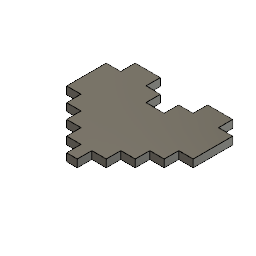
heart (Autodesk Fusion 360 design; units mm, degrees)
Autodesk Fusion 360 part; units mm, degrees
sketch "Sketch1" plane through (0, 0, 0) normal (0, 1, 0) x (1, 0, 0)
  line L0 (-2.775, 16.15) -> (-8.325, 16.15)
  line L1 (2.775, -22.7) -> (2.775, -17.15)
  line L2 (13.875, -11.6) -> (8.325, -11.6)
  line L3 (28.5, -28) -> (28.5, 27)
  line L4 (-2.775, -17.15) -> (-2.775, -22.7)
  line L5 (-2.775, -22.7) -> (2.775, -22.7)
  line L6 (8.325, -17.15) -> (2.775, -17.15)
  line L7 (-28.5, 27) -> (-28.5, -28)
  line L8 (28.5, 27) -> (-28.5, 27)
  line L9 (19.425, -6.05) -> (13.875, -6.05)
  line L10 (-8.325, -17.15) -> (-2.775, -17.15)
  line L11 (28.5, -0.5) -> (-28.5, -0.5)
  line L12 (24.975, -0.5) -> (19.425, -0.5)
  line L13 (19.425, -0.5) -> (19.425, -6.05)
  line L14 (-24.975, 16.15) -> (-24.975, -0.5)
  line L15 (0, 5.05) -> (0, -0.5)
  line L16 (-24.975, -0.5) -> (-19.425, -0.5)
  line L17 (0, 10.6) -> (-2.775, 10.6)
  line L18 (0, 27) -> (0, -28)
  line L19 (24.975, 16.15) -> (24.975, -0.5)
  line L20 (0, -0.5) -> (0, -22.7)
  line L21 (0, -0.5) -> (0, 21.7)
  line L22 (-13.875, -6.05) -> (-13.875, -11.6)
  line L23 (-19.425, -6.05) -> (-13.875, -6.05)
  line L24 (0, 10.6) -> (0, 5.05)
  line L25 (-19.425, -0.5) -> (-19.425, -6.05)
  line L26 (-8.325, -11.6) -> (-8.325, -17.15)
  line L27 (19.425, 21.7) -> (19.425, 16.15)
  line L28 (-19.425, 21.7) -> (-19.425, 16.15)
  line L29 (-13.875, -11.6) -> (-8.325, -11.6)
  line L30 (-8.325, 16.15) -> (-8.325, 21.7)
  line L31 (-2.775, 10.6) -> (-2.775, 16.15)
  line L32 (8.325, -11.6) -> (8.325, -17.15)
  line L33 (-28.5, -28) -> (28.5, -28)
  line L34 (13.875, -6.05) -> (13.875, -11.6)
  line L35 (0, 21.7) -> (0, 16.15)
  line L36 (19.425, 16.15) -> (24.975, 16.15)
  line L37 (0, 10.6) -> (2.775, 10.6)
  line L38 (2.775, 16.15) -> (8.325, 16.15)
  line L39 (2.775, 10.6) -> (2.775, 16.15)
  line L40 (8.325, 21.7) -> (19.425, 21.7)
  line L41 (8.325, 16.15) -> (8.325, 21.7)
  line L42 (-19.425, 16.15) -> (-24.975, 16.15)
  line L43 (-8.325, 21.7) -> (-19.425, 21.7)
  line L44 (0, 16.15) -> (0, 10.6)
  point P0 (0, -30)
  dimension "d1" = 22.2
  dimension "d2" = 22.2
  dimension "d3" = 5.55
  dimension "d4" = 5.55
  dimension "d5" = 2.775
  dimension "d6" = 2.775
  dimension "d7" = 5.55
  dimension "d8" = 5.55
  dimension "d9" = 5.55
  dimension "d10" = 5.55
  dimension "d11" = 11.1
  dimension "d12" = 11.1
  dimension "d13" = 5.55
  dimension "d14" = 5.55
  dimension "d15" = 5.55
  dimension "d16" = 5.55
  dimension "d17" = 16.65
  dimension "d18" = 16.65
  dimension "d19" = 5.55
  dimension "d20" = 5.55
  dimension "d21" = 5.55
  dimension "d22" = 5.55
  dimension "d23" = 5.55
  dimension "d24" = 5.55
  dimension "d25" = 5.55
  dimension "d26" = 5.55
  dimension "d27" = 5.55
  dimension "d28" = 5.55
  dimension "d29" = 5.55
  dimension "d30" = 5.55
  dimension "d31" = 5.55
  dimension "d32" = 5.55
  dimension "d33" = 5.55
  dimension "d34" = 5.55
  constraint midpoint L18.start L8
  constraint midpoint L18.end L33
  constraint midpoint L11.start L3
  constraint midpoint L11.end L7
  constraint midpoint L15.end L18
  constraint perpendicular L11 L21
  constraint parallel L18 L20
  constraint parallel L18 L35
  constraint parallel L18 L44
  constraint parallel L21 L24
  constraint parallel L15 L21
  constraint perpendicular L37 L44
  constraint perpendicular L17 L24
  constraint perpendicular L37 L39
  constraint perpendicular L38 L39
  constraint perpendicular L17 L31
  constraint perpendicular L0 L31
  constraint perpendicular L0 L30
  constraint perpendicular L38 L41
  constraint perpendicular L40 L41
  constraint perpendicular L30 L43
  constraint perpendicular L28 L43
  constraint perpendicular L27 L40
  constraint perpendicular L28 L42
  constraint perpendicular L27 L36
  constraint perpendicular L14 L42
  constraint perpendicular L19 L36
  constraint perpendicular L14 L16
  constraint perpendicular L12 L19
  constraint perpendicular L11 L13
  constraint perpendicular L16 L25
  constraint perpendicular L23 L25
  constraint perpendicular L9 L13
  constraint perpendicular L22 L23
  constraint perpendicular L9 L34
  constraint perpendicular L22 L29
  constraint perpendicular L2 L34
  constraint perpendicular L26 L29
  constraint perpendicular L2 L32
  constraint perpendicular L6 L32
  constraint perpendicular L10 L26
  constraint perpendicular L4 L10
  constraint perpendicular L5 L20
  measures "d1" distance of L15.end L21.end
  measures "d2" distance of L15.end L20.end
  measures "d3" distance of L15.start L17.start
  measures "d4" distance of L15.start L15.end
  measures "d5" distance of L37.end L17.start
  measures "d6" distance of L17.end L17.start
  measures "d7" distance of L37.end L38.start
  measures "d8" distance of L38.start L38.end
  measures "d9" distance of L17.end L0.start
  measures "d10" distance of L0.end L0.start
  measures "d11" distance of L40.start L27.start
  measures "d12" distance of L30.end L28.start
  measures "d13" distance of L28.end L28.start
  measures "d14" distance of L27.start L27.end
  measures "d15" distance of L28.end L14.start
  measures "d16" distance of L27.end L19.start
  measures "d17" distance of L14.start L14.end
  measures "d18" distance of L12.start L19.start
  measures "d19" distance of L16.end L14.end
  measures "d20" distance of L12.start L12.end
  measures "d21" distance of L9.start L12.end
  measures "d22" distance of L16.end L23.start
  measures "d23" distance of L23.start L22.start
  measures "d24" distance of L9.end L9.start
  measures "d25" distance of L22.end L22.start
  measures "d26" distance of L9.end L2.start
  measures "d27" distance of L26.start L22.end
  measures "d28" distance of L2.start L2.end
  measures "d29" distance of L26.start L10.start
  measures "d30" distance of L6.start L2.end
  measures "d31" distance of L6.start L1.end
  measures "d32" distance of L10.start L4.start
  measures "d33" distance of L4.end L4.start
  measures "d34" distance of L4.end L1.start
extrude "Extrude4" add sketch "Sketch1" along normal blind 3 contours L0 L11 L14 L15 L16 L17 L18 L21 L24 L28 L30 L31 L42 L43 | L11 L12 L15 L18 L19 L21 L24 L27 L36 L37 L38 L39 L40 L41 | L4 L5 L10 L11 L18 L20 L22 L23 L25 L26 L29 | L1 L2 L5 L6 L9 L11 L13 L18 L20 L32 L34
sketch "Sketch5" plane through (0, 3, 0) normal (0, 1, 0) x (-1, 0, 0)
  line L0 (-2.775, -10.6) -> (2.775, -10.6)
  line L1 (2.775, -10.6) -> (2.775, -16.15)
  line L2 (2.775, -16.15) -> (8.325, -16.15)
  line L3 (8.325, -16.15) -> (8.325, -21.7)
  line L4 (8.325, -21.7) -> (19.425, -21.7)
  line L5 (19.425, -21.7) -> (19.425, -16.15)
  line L6 (19.425, -16.15) -> (24.975, -16.15)
  line L7 (24.975, -16.15) -> (24.975, 0.5)
  line L8 (24.975, 0.5) -> (19.425, 0.5)
  line L9 (19.425, 0.5) -> (19.425, 6.05)
  line L10 (19.425, 6.05) -> (13.875, 6.05)
  line L11 (13.875, 6.05) -> (13.875, 11.6)
  line L12 (13.875, 11.6) -> (8.325, 11.6)
  line L13 (8.325, 11.6) -> (8.325, 17.15)
  line L14 (8.325, 17.15) -> (2.775, 17.15)
  line L15 (2.775, 17.15) -> (2.775, 22.7)
  line L16 (2.775, 22.7) -> (-2.775, 22.7)
  line L17 (-2.775, 22.7) -> (-2.775, 17.15)
  line L18 (-2.775, 17.15) -> (-8.325, 17.15)
  line L19 (-8.325, 17.15) -> (-8.325, 11.6)
  line L20 (-8.325, 11.6) -> (-13.875, 11.6)
  line L21 (-13.875, 11.6) -> (-13.875, 6.05)
  line L22 (-13.875, 6.05) -> (-19.425, 6.05)
  line L23 (-19.425, 6.05) -> (-19.425, 0.5)
  line L24 (-19.425, 0.5) -> (-24.975, 0.5)
  line L25 (-24.975, 0.5) -> (-24.975, -16.15)
  line L26 (-24.975, -16.15) -> (-19.425, -16.15)
  line L27 (-19.425, -16.15) -> (-19.425, -21.7)
  line L28 (-19.425, -21.7) -> (-8.325, -21.7)
  line L29 (-8.325, -21.7) -> (-8.325, -16.15)
  line L30 (-8.325, -16.15) -> (-2.775, -16.15)
  line L31 (-2.775, -16.15) -> (-2.775, -10.6)
  line L32 (-18.725, -15.45) -> (-18.725, -21)
  line L33 (-18.725, -21) -> (-9.025, -21)
  line L34 (-9.025, -21) -> (-9.025, -15.45)
  line L35 (-9.025, -15.45) -> (-3.475, -15.45)
  line L36 (-3.475, -15.45) -> (-3.475, -9.9)
  line L37 (-3.475, -9.9) -> (3.475, -9.9)
  line L38 (3.475, -9.9) -> (3.475, -15.45)
  line L39 (3.475, -15.45) -> (9.025, -15.45)
  line L40 (9.025, -15.45) -> (9.025, -21)
  line L41 (9.025, -21) -> (18.725, -21)
  line L42 (18.725, -21) -> (18.725, -15.45)
  line L43 (18.725, -15.45) -> (24.275, -15.45)
  line L44 (24.275, -15.45) -> (24.275, -0.2)
  line L45 (24.275, -0.2) -> (18.725, -0.2)
  line L46 (18.725, -0.2) -> (18.725, 5.35)
  line L47 (18.725, 5.35) -> (13.175, 5.35)
  line L48 (13.175, 5.35) -> (13.175, 10.9)
  line L49 (13.175, 10.9) -> (7.625, 10.9)
  line L50 (7.625, 10.9) -> (7.625, 16.45)
  line L51 (7.625, 16.45) -> (2.075, 16.45)
  line L52 (2.075, 16.45) -> (2.075, 22)
  line L53 (2.075, 22) -> (-2.075, 22)
  line L54 (-2.075, 22) -> (-2.075, 16.45)
  line L55 (-2.075, 16.45) -> (-7.625, 16.45)
  line L56 (-7.625, 16.45) -> (-7.625, 10.9)
  line L57 (-7.625, 10.9) -> (-13.175, 10.9)
  line L58 (-13.175, 10.9) -> (-13.175, 5.35)
  line L59 (-13.175, 5.35) -> (-18.725, 5.35)
  line L60 (-18.725, 5.35) -> (-18.725, -0.2)
  line L61 (-18.725, -0.2) -> (-24.275, -0.2)
  line L62 (-24.275, -0.2) -> (-24.275, -15.45)
  line L63 (-24.275, -15.45) -> (-18.725, -15.45)
  dimension "d53" = -0.7
extrude "Extrude8" cut sketch "Sketch5" against normal blind 25
equation "d1 = ( 44.4 / 2 ) * 1 mm"
equation "d2 = ( 44.4 / 2 ) * 1 mm"
equation "d5 = ( 5.55 / 2 ) * 1 mm"
equation "d6 = ( 5.55 / 2 ) * 1 mm"
equation "d11 = ( 5.55 * 2 ) * 1 mm"
equation "d12 = ( 5.55 * 2 ) * 1 mm"
equation "d17 = ( 5.55 * 3 ) * 1 mm"
equation "d18 = ( 5.55 * 3 ) * 1 mm"
